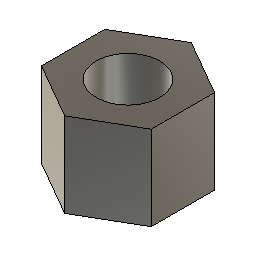
Hex Bolt Spacers v5 (Autodesk Fusion 360 design; units mm, degrees)
Autodesk Fusion 360 part; units mm, degrees
sketch "Sketch1" plane through (0, 0, 0) normal (0, 0, 1) x (1, 0, 0)
  circle A0 centre (0, 0) radius 9.525 construction
  line L0 (0, 0) -> (0, 9.525) construction
  line L1 (0, 0) -> (8.2489, -4.7625) construction
  line L2 (0, 0) -> (-8.2489, -4.7625) construction
  line L3 (0, 0) -> (0, -9.525) construction
  line L4 (0, 0) -> (-8.2489, 4.7625) construction
  line L5 (0, 0) -> (8.2489, 4.7625) construction
  line L6 (-8.2489, 4.7625) -> (0, 9.525)
  line L7 (0, 9.525) -> (8.2489, 4.7625)
  line L8 (8.2489, 4.7625) -> (8.2489, -4.7625)
  line L9 (8.2489, -4.7625) -> (0, -9.525)
  line L10 (-8.2489, -4.7625) -> (0, -9.525)
  line L11 (-8.2489, 4.7625) -> (-8.2489, -4.7625)
  circle A1 centre (0, 0) radius 4.7625
  dimension "d1" = 19.05
  constraint coincident A0.centre L0.start
  constraint coincident A0 L0.end
  constraint vertical L0
  constraint coincident A0 L1.end
  constraint coincident A0 L3.end
  constraint vertical L3
  constraint coincident A0 L4.end
  constraint parallel L1 L4
  constraint coincident A0 L5.end
  constraint parallel L2 L5
  constraint vertical L8
  constraint parallel L7 L10
  measures "d1" diameter of A0
extrude "Extrude1" add sketch "Sketch1" along normal blind 12.7
sketch "Sketch2" plane through (0, 0, 12.7) normal (0, 0, 1) x (-1, 0, 0)
  circle A0 centre (0, 0) radius 4.7625
  line L0 (0, -9.525) -> (8.2489, -4.7625)
  line L1 (8.2489, -4.7625) -> (8.2489, 4.7625)
  line L2 (8.2489, 4.7625) -> (0, 9.525)
  line L3 (0, 9.525) -> (-8.2489, 4.7625)
  line L4 (-8.2489, 4.7625) -> (-8.2489, -4.7625)
  line L5 (-8.2489, -4.7625) -> (0, -9.525)
